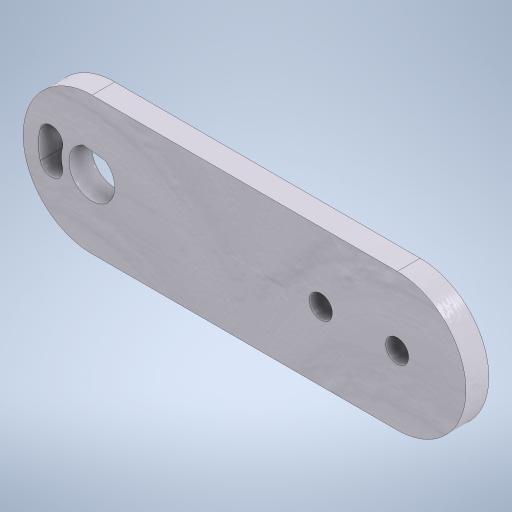
# Autodesk Inventor part: Arm2
Saved by Autodesk Inventor 2023 (Build 270158000, 158)
## iProperties
Created: 2024-02-05
Part Number: Arm2
Material: Aluminum 6061, Welded
Document SubType Name: Modeling
Designer: victo
Density: 2.7 g/cm^3
Appearance: Weld - Aluminum
Author: victo
Autodesk Inventor part; units mm, degrees
ref_plane "YZ Plane" through (0, 0, 0) normal (1, 0, 0) x (0, 1, 0)
ref_plane "XZ Plane" through (0, 0, 0) normal (0, 1, 0) x (-1, 0, 0)
ref_plane "XY Plane" through (0, 0, 0) normal (0, 0, 1) x (1, 0, 0)
sketch "Sketch1" plane through (0, 0, 0) normal (0, 0, 1) x (1, 0, 0)
  circle A0 centre (0, 0) radius 3
  line L0 (0, 0) -> (40, 0) construction
  line L1 (0, -9) -> (40, -9)
  line L2 (40, 9) -> (0, 9)
  arc A1 (0, 9) -> (0, -9) centre (0, 0) ccw
  arc A2 (40, -9) -> (40, 9) centre (40, 0) ccw
  line L3 (0, 0) -> (40, 0) construction
  circle A3 centre (40, 0) radius 1.5
  circle A4 centre (30, 0) radius 1.5
  circle A5 centre (-5.3126, -1.4235) radius 1.5
  circle A6 centre (-5.3126, 1.4235) radius 1.5
  line L4 (0, 0) -> (-5.3126, 1.4235) construction
  line L5 (0, 0) -> (-5.3126, -1.4235) construction
  line L6 (0, 0) -> (-9, 0) construction
  arc A7 (-3.8637, 1.0353) -> (-3.8637, -1.0353) centre (0, 0) ccw
  arc A8 (-6.7617, 1.811) -> (-6.7615, -1.8117) centre (0, 0) ccw
  line L7 (-1.158, 2.7675) -> (1.7295, 2.4513)
  point P0 (20, 0)
  dimension "d0" = 6
  dimension "d1" = 40
  dimension "d2" = 0
  dimension "d3" = 18
  dimension "d4" = 3
  dimension "d5" = 3
  dimension "d6" = 10
  dimension "d7" = 3
  dimension "d8" = 3
  dimension "d9" = 15
  dimension "d10" = 15
  dimension "d11" = 5.5
  dimension "d12" = 5.5
  dimension "d15" = 2.625
  dimension "d16" = 6.25
  constraints: 18 end point, 15 point on circle, 9 centre point, 6 tangent, 4 coincident, 2 horizontal, 1 collinear, 1 midpoint, 1 parallel, 1 point on line
  measures "d0" diameter of A0
  measures "d1" distance of L0.start L0.end
  measures "d2" distance between parallel lines of L0 L3
  measures "d3" diameter of A2
  measures "d4" diameter of A3
  measures "d5" diameter of A4
  measures "d6" distance of A4.centre L0.end
  measures "d7" diameter of A5
  measures "d8" diameter of A6
  measures "d9" angle of L5 L6
  measures "d10" angle of L6 L4
  measures "d11" distance of L0.start L4.end
  measures "d12" distance of L0.start L5.end
  measures "d15" distance from line of L7 point (0, 0)
  measures "d16" angle of L0 L7
extrude "Extrusion1" add sketch "Sketch1" along normal blind 3 contours L7 A0 | A1 L2 A2 L1 picked at (0.1985, 2.7396)
body "Solid1"
